Autodesk Fusion 360 part; units mm, degrees
(part 9 of 11)
  spline S8 degree 5 poles (-23.7664, -79.2655) (-23.7765, -79.2987) (-23.7959, -79.3651) (-23.8224, -79.4654) (-23.8532, -79.6002) (-23.8854, -79.7703) (-23.913, -79.9414) (-23.9379, -80.1132) (-23.9612, -80.2854) (-23.9836, -80.4578) (-24.0048, -80.6305) (-24.0246, -80.8034) (-24.0425, -80.9767) (-24.0582, -81.1505) (-24.0717, -81.3247) (-24.0832, -81.4994) (-24.0929, -81.6743) (-24.1011, -81.8495) (-24.1081, -82.0249) (-24.1139, -82.2005) (-24.1185, -82.3763) (-24.1218, -82.5523) (-24.1237, -82.7285) (-24.1243, -82.905) (-24.1235, -83.0816) (-24.1214, -83.2584) (-24.1181, -83.4354) (-24.1136, -83.6125) (-24.108, -83.7898) (-24.1013, -83.9672) (-24.0934, -84.1448) (-24.0845, -84.3225) (-24.0745, -84.5003) (-24.0634, -84.6782) (-24.0512, -84.8563) (-24.0379, -85.0344) (-24.0236, -85.2127) (-24.0082, -85.391) (-23.9919, -85.5695) (-23.9746, -85.748) (-23.9562, -85.9266) (-23.9369, -86.1053) (-23.9167, -86.2841) (-23.8955, -86.4629) (-23.8733, -86.6418) (-23.8502, -86.8207) (-23.8261, -86.9998) (-23.8011, -87.1788) (-23.7753, -87.3579) (-23.7485, -87.5371) (-23.7208, -87.7163) (-23.6922, -87.8956) (-23.6628, -88.0748) (-23.6324, -88.2541) (-23.6012, -88.4335) (-23.5692, -88.6129) (-23.5362, -88.7922) (-23.5025, -88.9717) (-23.4679, -89.1511) (-23.4324, -89.3305) (-23.3961, -89.51) (-23.359, -89.6894) (-23.3211, -89.8689) (-23.2823, -90.0484) (-23.2428, -90.2278) (-23.2024, -90.4073) (-23.1613, -90.5868) (-23.1193, -90.7662) (-23.0766, -90.9456) (-23.033, -91.1251) (-22.9887, -91.3045) (-22.9527, -91.448) (-22.9253, -91.5556) (-22.9068, -91.6274) (-22.8976, -91.6633) knots 0 0 0 0 0 0 0.01428571 0.02857143 0.04285714 0.05714286 0.07142857 0.08571429 0.1 0.11428571 0.12857143 0.14285714 0.15714286 0.17142857 0.18571429 0.2 0.21428571 0.22857143 0.24285714 0.25714286 0.27142857 0.28571429 0.3 0.31428571 0.32857143 0.34285714 0.35714286 0.37142857 0.38571429 0.4 0.41428571 0.42857143 0.44285714 0.45714286 0.47142857 0.48571429 0.5 0.51428571 0.52857143 0.54285714 0.55714286 0.57142857 0.58571429 0.6 0.61428571 0.62857143 0.64285714 0.65714286 0.67142857 0.68571429 0.7 0.71428571 0.72857143 0.74285714 0.75714286 0.77142857 0.78571429 0.8 0.81428571 0.82857143 0.84285714 0.85714286 0.87142857 0.88571429 0.9 0.91428571 0.92857143 0.94285714 0.95714286 0.97142857 0.98571429 1 1 1 1 1 1
  arc A22 (-22.8976, -91.6633) -> (-18.3724, -92.6961) centre (0.5538, 0.6546) ccw
  spline S9 degree 5 poles (-12.2104, -81.9031) (-12.2157, -81.9373) (-12.2271, -82.0056) (-12.2467, -82.1075) (-12.2774, -82.2423) (-12.3222, -82.4095) (-12.3716, -82.5757) (-12.4237, -82.7413) (-12.4774, -82.9065) (-12.5321, -83.0716) (-12.5879, -83.2363) (-12.645, -83.4007) (-12.7041, -83.5647) (-12.7654, -83.728) (-12.8288, -83.8909) (-12.8942, -84.0532) (-12.9614, -84.215) (-13.03, -84.3764) (-13.0998, -84.5375) (-13.1708, -84.6982) (-13.243, -84.8586) (-13.3164, -85.0186) (-13.3911, -85.1782) (-13.4671, -85.3374) (-13.5444, -85.4962) (-13.623, -85.6546) (-13.7028, -85.8126) (-13.7837, -85.9703) (-13.8657, -86.1276) (-13.9487, -86.2845) (-14.0328, -86.4411) (-14.118, -86.5973) (-14.2041, -86.7531) (-14.2914, -86.9086) (-14.3796, -87.0637) (-14.4689, -87.2185) (-14.5591, -87.3729) (-14.6503, -87.5269) (-14.7425, -87.6806) (-14.8355, -87.8339) (-14.9295, -87.9869) (-15.0244, -88.1395) (-15.1203, -88.2918) (-15.217, -88.4437) (-15.3146, -88.5953) (-15.4131, -88.7465) (-15.5124, -88.8973) (-15.6126, -89.0478) (-15.7136, -89.198) (-15.8155, -89.3478) (-15.9182, -89.4972) (-16.0217, -89.6463) (-16.126, -89.795) (-16.2312, -89.9434) (-16.3371, -90.0915) (-16.4438, -90.2392) (-16.5513, -90.3865) (-16.6596, -90.5335) (-16.7686, -90.6801) (-16.8784, -90.8264) (-16.9889, -90.9724) (-17.1002, -91.118) (-17.2123, -91.2632) (-17.3251, -91.4081) (-17.4386, -91.5526) (-17.5528, -91.6968) (-17.6677, -91.8406) (-17.7834, -91.9841) (-17.8998, -92.1272) (-18.0168, -92.27) (-18.1346, -92.4124) (-18.2294, -92.5261) (-18.3008, -92.6111) (-18.3485, -92.6678) (-18.3724, -92.6961) knots 0 0 0 0 0 0 0.01428571 0.02857143 0.04285714 0.05714286 0.07142857 0.08571429 0.1 0.11428571 0.12857143 0.14285714 0.15714286 0.17142857 0.18571429 0.2 0.21428571 0.22857143 0.24285714 0.25714286 0.27142857 0.28571429 0.3 0.31428571 0.32857143 0.34285714 0.35714286 0.37142857 0.38571429 0.4 0.41428571 0.42857143 0.44285714 0.45714286 0.47142857 0.48571429 0.5 0.51428571 0.52857143 0.54285714 0.55714286 0.57142857 0.58571429 0.6 0.61428571 0.62857143 0.64285714 0.65714286 0.67142857 0.68571429 0.7 0.71428571 0.72857143 0.74285714 0.75714286 0.77142857 0.78571429 0.8 0.81428571 0.82857143 0.84285714 0.85714286 0.87142857 0.88571429 0.9 0.91428571 0.92857143 0.94285714 0.95714286 0.97142857 0.98571429 1 1 1 1 1 1
  line L9 (-12.2104, -81.9031) -> (-11.9819, -80.4264)
  arc A23 (-11.0838, -79.7623) -> (-11.9819, -80.4264) centre (-11.1974, -80.5478) ccw
  arc A24 (-11.0838, -79.7623) -> (-5.9948, -80.3356) centre (0.5538, 0.6546) ccw
  arc A25 (-5.267, -81.183) -> (-5.9948, -80.3356) centre (-6.0588, -81.1268) ccw
  line L10 (-5.267, -81.183) -> (-5.3728, -82.6735)
  spline S10 degree 5 poles (-5.3728, -82.6735) (-5.3752, -82.7081) (-5.3793, -82.7772) (-5.3829, -82.8808) (-5.3829, -83.0191) (-5.3764, -83.1921) (-5.3653, -83.3651) (-5.3513, -83.5381) (-5.3357, -83.7112) (-5.3191, -83.8843) (-5.3014, -84.0573) (-5.2823, -84.2303) (-5.2612, -84.4033) (-5.2378, -84.5762) (-5.2122, -84.749) (-5.1845, -84.9218) (-5.155, -85.0946) (-5.1241, -85.2672) (-5.0918, -85.4398) (-5.0584, -85.6123) (-5.0237, -85.7847) (-4.9878, -85.957) (-4.9505, -86.1292) (-4.9118, -86.3013) (-4.8717, -86.4734) (-4.8304, -86.6453) (-4.7877, -86.8171) (-4.7439, -86.9888) (-4.699, -87.1604) (-4.653, -87.3319) (-4.6058, -87.5032) (-4.5576, -87.6745) (-4.5082, -87.8456) (-4.4578, -88.0166) (-4.4063, -88.1874) (-4.3537, -88.3582) (-4.3001, -88.5288) (-4.2454, -88.6993) (-4.1898, -88.8696) (-4.1332, -89.0398) (-4.0756, -89.2098) (-4.017, -89.3798) (-3.9575, -89.5495) (-3.897, -89.7191) (-3.8356, -89.8886) (-3.7732, -90.058) (-3.7099, -90.2271) (-3.6457, -90.3962) (-3.5806, -90.565) (-3.5147, -90.7337) (-3.4478, -90.9023) (-3.3801, -91.0707) (-3.3114, -91.2389) (-3.242, -91.407) (-3.1716, -91.5749) (-3.1005, -91.7426) (-3.0285, -91.9102) (-2.9556, -92.0776) (-2.8819, -92.2448) (-2.8074, -92.4119) (-2.7321, -92.5787) (-2.656, -92.7454) (-2.5791, -92.912) (-2.5014, -93.0783) (-2.4229, -93.2445) (-2.3436, -93.4105) (-2.2636, -93.5763) (-2.1827, -93.7419) (-2.1011, -93.9073) (-2.0188, -94.0725) (-1.9356, -94.2376) (-1.8685, -94.3695) (-1.8179, -94.4683) (-1.7839, -94.5342) (-1.7669, -94.5671) knots 0 0 0 0 0 0 0.01428571 0.02857143 0.04285714 0.05714286 0.07142857 0.08571429 0.1 0.11428571 0.12857143 0.14285714 0.15714286 0.17142857 0.18571429 0.2 0.21428571 0.22857143 0.24285714 0.25714286 0.27142857 0.28571429 0.3 0.31428571 0.32857143 0.34285714 0.35714286 0.37142857 0.38571429 0.4 0.41428571 0.42857143 0.44285714 0.45714286 0.47142857 0.48571429 0.5 0.51428571 0.52857143 0.54285714 0.55714286 0.57142857 0.58571429 0.6 0.61428571 0.62857143 0.64285714 0.65714286 0.67142857 0.68571429 0.7 0.71428571 0.72857143 0.74285714 0.75714286 0.77142857 0.78571429 0.8 0.81428571 0.82857143 0.84285714 0.85714286 0.87142857 0.88571429 0.9 0.91428571 0.92857143 0.94285714 0.95714286 0.97142857 0.98571429 1 1 1 1 1 1
  arc A26 (-1.7669, -94.5671) -> (2.8746, -94.5671) centre (0.5538, 0.6546) ccw
  spline S11 degree 5 poles (6.4805, -82.6735) (6.4829, -82.7081) (6.487, -82.7772) (6.4906, -82.8808) (6.4906, -83.0191) (6.4841, -83.1921) (6.473, -83.3651) (6.459, -83.5381) (6.4434, -83.7112) (6.4268, -83.8843) (6.4091, -84.0573) (6.39, -84.2303) (6.3689, -84.4033) (6.3455, -84.5762) (6.3199, -84.749) (6.2922, -84.9218) (6.2627, -85.0946) (6.2318, -85.2672) (6.1995, -85.4398) (6.1661, -85.6123) (6.1314, -85.7847) (6.0955, -85.957) (6.0582, -86.1292) (6.0195, -86.3013) (5.9794, -86.4734) (5.9381, -86.6453) (5.8954, -86.8171) (5.8516, -86.9888) (5.8067, -87.1604) (5.7607, -87.3319) (5.7135, -87.5032) (5.6653, -87.6745) (5.6159, -87.8456) (5.5655, -88.0166) (5.514, -88.1874) (5.4614, -88.3582) (5.4078, -88.5288) (5.3531, -88.6993) (5.2975, -88.8696) (5.2409, -89.0398) (5.1833, -89.2098) (5.1247, -89.3798) (5.0652, -89.5495) (5.0047, -89.7191) (4.9432, -89.8886) (4.8809, -90.058) (4.8176, -90.2271) (4.7534, -90.3962) (4.6883, -90.565) (4.6223, -90.7337) (4.5555, -90.9023) (4.4877, -91.0707) (4.4191, -91.2389) (4.3497, -91.407) (4.2793, -91.5749) (4.2082, -91.7426) (4.1361, -91.9102) (4.0633, -92.0776) (3.9896, -92.2448) (3.9151, -92.4119) (3.8398, -92.5787) (3.7637, -92.7454) (3.6868, -92.912) (3.6091, -93.0783) (3.5306, -93.2445) (3.4513, -93.4105) (3.3712, -93.5763) (3.2904, -93.7419) (3.2088, -93.9073) (3.1264, -94.0725) (3.0433, -94.2376) (2.9762, -94.3695) (2.9255, -94.4683) (2.8916, -94.5342) (2.8746, -94.5671) knots 0 0 0 0 0 0 0.01428571 0.02857143 0.04285714 0.05714286 0.07142857 0.08571429 0.1 0.11428571 0.12857143 0.14285714 0.15714286 0.17142857 0.18571429 0.2 0.21428571 0.22857143 0.24285714 0.25714286 0.27142857 0.28571429 0.3 0.31428571 0.32857143 0.34285714 0.35714286 0.37142857 0.38571429 0.4 0.41428571 0.42857143 0.44285714 0.45714286 0.47142857 0.48571429 0.5 0.51428571 0.52857143 0.54285714 0.55714286 0.57142857 0.58571429 0.6 0.61428571 0.62857143 0.64285714 0.65714286 0.67142857 0.68571429 0.7 0.71428571 0.72857143 0.74285714 0.75714286 0.77142857 0.78571429 0.8 0.81428571 0.82857143 0.84285714 0.85714286 0.87142857 0.88571429 0.9 0.91428571 0.92857143 0.94285714 0.95714286 0.97142857 0.98571429 1 1 1 1 1 1
  line L11 (6.4805, -82.6735) -> (6.3747, -81.183)
  arc A27 (7.1025, -80.3356) -> (6.3747, -81.183) centre (7.1664, -81.1268) ccw
  arc A28 (7.1025, -80.3356) -> (12.1914, -79.7623) centre (0.5538, 0.6546) ccw
  arc A29 (13.0895, -80.4264) -> (12.1914, -79.7623) centre (12.3051, -80.5478) ccw
  line L12 (13.0895, -80.4264) -> (13.3181, -81.9031)
  spline S12 degree 5 poles (13.3181, -81.9031) (13.3234, -81.9373) (13.3348, -82.0056) (13.3544, -82.1075) (13.3851, -82.2423) (13.4299, -82.4095) (13.4793, -82.5757) (13.5314, -82.7413) (13.5851, -82.9065) (13.6398, -83.0716) (13.6955, -83.2363) (13.7527, -83.4007) (13.8118, -83.5647) (13.873, -83.728) (13.9365, -83.8909) (14.0019, -84.0532) (14.0691, -84.215) (14.1377, -84.3764) (14.2075, -84.5375) (14.2785, -84.6982) (14.3507, -84.8586) (14.424, -85.0186) (14.4987, -85.1782) (14.5748, -85.3374) (14.6521, -85.4962) (14.7307, -85.6546) (14.8105, -85.8126) (14.8914, -85.9703) (14.9734, -86.1276) (15.0564, -86.2845) (15.1405, -86.4411) (15.2256, -86.5973) (15.3118, -86.7531) (15.399, -86.9086) (15.4873, -87.0637) (15.5766, -87.2185) (15.6668, -87.3729) (15.758, -87.5269) (15.8501, -87.6806) (15.9432, -87.8339) (16.0372, -87.9869) (16.1321, -88.1395) (16.2279, -88.2918) (16.3247, -88.4437) (16.4223, -88.5953) (16.5207, -88.7465) (16.6201, -88.8973) (16.7203, -89.0478) (16.8213, -89.198) (16.9232, -89.3478) (17.0259, -89.4972) (17.1294, -89.6463) (17.2337, -89.795) (17.3388, -89.9434) (17.4448, -90.0915) (17.5515, -90.2392) (17.659, -90.3865) (17.7672, -90.5335) (17.8763, -90.6801) (17.9861, -90.8264) (18.0966, -90.9724) (18.2079, -91.118) (18.32, -91.2632) (18.4327, -91.4081) (18.5462, -91.5526) (18.6605, -91.6968) (18.7754, -91.8406) (18.8911, -91.9841) (19.0075, -92.1272) (19.1245, -92.27) (19.2423, -92.4124) (19.3371, -92.5261) (19.4084, -92.6111) (19.4562, -92.6678) (19.4801, -92.6961) knots 0 0 0 0 0 0 0.01428571 0.02857143 0.04285714 0.05714286 0.07142857 0.08571429 0.1 0.11428571 0.12857143 0.14285714 0.15714286 0.17142857 0.18571429 0.2 0.21428571 0.22857143 0.24285714 0.25714286 0.27142857 0.28571429 0.3 0.31428571 0.32857143 0.34285714 0.35714286 0.37142857 0.38571429 0.4 0.41428571 0.42857143 0.44285714 0.45714286 0.47142857 0.48571429 0.5 0.51428571 0.52857143 0.54285714 0.55714286 0.57142857 0.58571429 0.6 0.61428571 0.62857143 0.64285714 0.65714286 0.67142857 0.68571429 0.7 0.71428571 0.72857143 0.74285714 0.75714286 0.77142857 0.78571429 0.8 0.81428571 0.82857143 0.84285714 0.85714286 0.87142857 0.88571429 0.9 0.91428571 0.92857143 0.94285714 0.95714286 0.97142857 0.98571429 1 1 1 1 1 1
  arc A30 (19.4801, -92.6961) -> (24.0053, -91.6633) centre (0.5538, 0.6546) ccw
  spline S13 degree 5 poles (24.8741, -79.2655) (24.8842, -79.2987) (24.9035, -79.3651) (24.9301, -79.4654) (24.9609, -79.6002) (24.9931, -79.7703) (25.0207, -79.9414) (25.0456, -80.1132) (25.0689, -80.2854) (25.0912, -80.4578) (25.1125, -80.6305) (25.1323, -80.8034) (25.1502, -80.9767) (25.1659, -81.1505) (25.1794, -81.3247) (25.1909, -81.4994) (25.2006, -81.6743) (25.2088, -81.8495) (25.2158, -82.0249) (25.2216, -82.2005) (25.2261, -82.3763) (25.2294, -82.5523) (25.2314, -82.7285) (25.232, -82.905) (25.2312, -83.0816) (25.2291, -83.2584) (25.2258, -83.4354) (25.2213, -83.6125) (25.2157, -83.7898) (25.209, -83.9672) (25.2011, -84.1448) (25.1922, -84.3225) (25.1822, -84.5003) (25.171, -84.6782) (25.1588, -84.8563) (25.1456, -85.0344) (25.1312, -85.2127) (25.1159, -85.391) (25.0996, -85.5695) (25.0822, -85.748) (25.0639, -85.9266) (25.0446, -86.1053) (25.0244, -86.2841) (25.0031, -86.4629) (24.981, -86.6418) (24.9578, -86.8207) (24.9338, -86.9998) (24.9088, -87.1788) (24.8829, -87.3579) (24.8562, -87.5371) (24.8285, -87.7163) (24.7999, -87.8956) (24.7705, -88.0748) (24.7401, -88.2541) (24.7089, -88.4335) (24.6769, -88.6129) (24.6439, -88.7922) (24.6102, -88.9717) (24.5755, -89.1511) (24.5401, -89.3305) (24.5038, -89.51) (24.4667, -89.6894) (24.4288, -89.8689) (24.39, -90.0484) (24.3505, -90.2278) (24.3101, -90.4073) (24.2689, -90.5868) (24.227, -90.7662) (24.1843, -90.9456) (24.1407, -91.1251) (24.0964, -91.3045) (24.0603, -91.448) (24.0329, -91.5556) (24.0145, -91.6274) (24.0053, -91.6633) knots 0 0 0 0 0 0 0.01428571 0.02857143 0.04285714 0.05714286 0.07142857 0.08571429 0.1 0.11428571 0.12857143 0.14285714 0.15714286 0.17142857 0.18571429 0.2 0.21428571 0.22857143 0.24285714 0.25714286 0.27142857 0.28571429 0.3 0.31428571 0.32857143 0.34285714 0.35714286 0.37142857 0.38571429 0.4 0.41428571 0.42857143 0.44285714 0.45714286 0.47142857 0.48571429 0.5 0.51428571 0.52857143 0.54285714 0.55714286 0.57142857 0.58571429 0.6 0.61428571 0.62857143 0.64285714 0.65714286 0.67142857 0.68571429 0.7 0.71428571 0.72857143 0.74285714 0.75714286 0.77142857 0.78571429 0.8 0.81428571 0.82857143 0.84285714 0.85714286 0.87142857 0.88571429 0.9 0.91428571 0.92857143 0.94285714 0.95714286 0.97142857 0.98571429 1 1 1 1 1 1
  line L13 (24.8741, -79.2655) -> (24.4393, -77.8359)
  arc A31 (24.9603, -76.8478) -> (24.4393, -77.8359) centre (25.1987, -77.6049) ccw
  arc A32 (24.9603, -76.8478) -> (29.7941, -75.1564) centre (0.5538, 0.6546) ccw
  arc A33 (30.8175, -75.6041) -> (29.7941, -75.1564) centre (30.0797, -75.897) ccw
  line L14 (30.8175, -75.6041) -> (31.3689, -76.9929)
  spline S14 degree 5 poles (31.3689, -76.9929) (31.3817, -77.0251) (31.408, -77.0891) (31.4497, -77.1841) (31.5097, -77.3087) (31.5906, -77.4617) (31.6757, -77.6127) (31.7634, -77.7626) (31.8525, -77.9118) (31.9425, -78.0605) (32.0336, -78.2087) (32.1259, -78.3563) (32.2199, -78.5029) (32.316, -78.6486) (32.4141, -78.7932) (32.514, -78.9369) (32.6155, -79.0797) (32.7183, -79.2218) (32.8222, -79.3633) (32.9272, -79.5042) (33.0332, -79.6445) (33.1404, -79.7842) (33.2487, -79.9232) (33.3583, -80.0615) (33.469, -80.1991) (33.5809, -80.336) (33.6938, -80.4723) (33.8078, -80.608) (33.9227, -80.7431) (34.0386, -80.8776) (34.1554, -81.0116) (34.2732, -81.1449) (34.3919, -81.2777) (34.5115, -81.4098) (34.6321, -81.5414) (34.7535, -81.6724) (34.8758, -81.8029) (34.999, -81.9328) (35.1231, -82.0621) (35.2479, -82.1909) (35.3736, -82.3191) (35.5001, -82.4468) (35.6274, -82.5739) (35.7555, -82.7005) (35.8844, -82.8265) (36.014, -82.952) (36.1444, -83.077) (36.2756, -83.2014) (36.4075, -83.3253) (36.5402, -83.4487) (36.6735, -83.5715) (36.8076, -83.6939) (36.9425, -83.8157) (37.078, -83.9369) (37.2142, -84.0577) (37.3511, -84.178) (37.4887, -84.2977) (37.6269, -84.4169) (37.7659, -84.5356) (37.9055, -84.6538) (38.0457, -84.7715) (38.1866, -84.8886) (38.3282, -85.0053) (38.4704, -85.1214) (38.6132, -85.2371) (38.7566, -85.3522) (38.9007, -85.4669) (39.0454, -85.581) (39.1907, -85.6947) (39.3366, -85.8078) (39.4831, -85.9205) (39.6008, -86.0102) (39.6893, -86.0772) (39.7485, -86.1218) (39.7781, -86.1441) knots 0 0 0 0 0 0 0.01428571 0.02857143 0.04285714 0.05714286 0.07142857 0.08571429 0.1 0.11428571 0.12857143 0.14285714 0.15714286 0.17142857 0.18571429 0.2 0.21428571 0.22857143 0.24285714 0.25714286 0.27142857 0.28571429 0.3 0.31428571 0.32857143 0.34285714 0.35714286 0.37142857 0.38571429 0.4 0.41428571 0.42857143 0.44285714 0.45714286 0.47142857 0.48571429 0.5 0.51428571 0.52857143 0.54285714 0.55714286 0.57142857 0.58571429 0.6 0.61428571 0.62857143 0.64285714 0.65714286 0.67142857 0.68571429 0.7 0.71428571 0.72857143 0.74285714 0.75714286 0.77142857 0.78571429 0.8 0.81428571 0.82857143 0.84285714 0.85714286 0.87142857 0.88571429 0.9 0.91428571 0.92857143 0.94285714 0.95714286 0.97142857 0.98571429 1 1 1 1 1 1
  arc A34 (39.7781, -86.1441) -> (43.9599, -84.1302) centre (0.5538, 0.6546) ccw
  spline S15 degree 5 poles (42.0483, -71.85) (42.0655, -71.88) (42.0991, -71.9405) (42.1473, -72.0324) (42.2074, -72.157) (42.2766, -72.3156) (42.3416, -72.4763) (42.4041, -72.6383) (42.4651, -72.801) (42.5253, -72.9641) (42.5844, -73.1277) (42.6422, -73.2919) (42.6982, -73.4569) (42.7522, -73.6228) (42.8041, -73.7896) (42.8542, -73.9573) (42.9025, -74.1257) (42.9496, -74.2947) (42.9954, -74.4642) (43.0401, -74.6341) (43.0837, -74.8045) (43.1261, -74.9753) (43.1672, -75.1467) (43.207, -75.3185) (43.2456, -75.4909) (43.2829, -75.6638) (43.319, -75.8371) (43.354, -76.0108) (43.388, -76.1848) (43.4209, -76.3593) (43.4528, -76.5342) (43.4836, -76.7094) (43.5134, -76.885) (43.5422, -77.0609) (43.5699, -77.2372) (43.5966, -77.4138) (43.6223, -77.5908) (43.6471, -77.7681) (43.6708, -77.9457) (43.6937, -78.1236) (43.7155, -78.3018) (43.7365, -78.4803) (43.7565, -78.6591) (43.7756, -78.8382) (43.7938, -79.0175) (43.8111, -79.1971) (43.8275, -79.377) (43.843, -79.5572) (43.8576, -79.7375) (43.8714, -79.9182) (43.8842, -80.0991) (43.8963, -80.2802) (43.9075, -80.4615) (43.9178, -80.6431) (43.9273, -80.8249) (43.9359, -81.0069) (43.9437, -81.1891) (43.9507, -81.3715) (43.9569, -81.5541) (43.9623, -81.737) (43.9669, -81.92) (43.9706, -82.1032) (43.9736, -82.2866) (43.9757, -82.4702) (43.9771, -82.654) (43.9777, -82.8379) (43.9775, -83.022) (43.9765, -83.2063) (43.9748, -83.3908) (43.9723, -83.5754) (43.969, -83.7602) (43.9657, -83.9081) (43.963, -84.0191) (43.961, -84.0932) (43.9599, -84.1302) knots 0 0 0 0 0 0 0.01428571 0.02857143 0.04285714 0.05714286 0.07142857 0.08571429 0.1 0.11428571 0.12857143 0.14285714 0.15714286 0.17142857 0.18571429 0.2 0.21428571 0.22857143 0.24285714 0.25714286 0.27142857 0.28571429 0.3 0.31428571 0.32857143 0.34285714 0.35714286 0.37142857 0.38571429 0.4 0.41428571 0.42857143 0.44285714 0.45714286 0.47142857 0.48571429 0.5 0.51428571 0.52857143 0.54285714 0.55714286 0.57142857 0.58571429 0.6 0.61428571 0.62857143 0.64285714 0.65714286 0.67142857 0.68571429 0.7 0.71428571 0.72857143 0.74285714 0.75714286 0.77142857 0.78571429 0.8 0.81428571 0.82857143 0.84285714 0.85714286 0.87142857 0.88571429 0.9 0.91428571 0.92857143 0.94285714 0.95714286 0.97142857 0.98571429 1 1 1 1 1 1
  line L15 (42.0483, -71.85) -> (41.3063, -70.553)
  arc A35 (41.5943, -69.4737) -> (41.3063, -70.553) centre (41.9952, -70.1588) ccw
  arc A36 (41.5943, -69.4737) -> (45.9305, -66.7491) centre (0.5538, 0.6546) ccw
  arc A37 (47.0279, -66.9578) -> (45.9305, -66.7491) centre (46.3738, -67.4076) ccw
  line L16 (47.0279, -66.9578) -> (47.8745, -68.1891)
  spline S16 degree 5 poles (47.8745, -68.1891) (47.8941, -68.2177) (47.934, -68.2742) (47.9958, -68.3575) (48.082, -68.4657) (48.1949, -68.5968) (48.3115, -68.7252) (48.4304, -68.8517) (48.5504, -68.9773) (48.6713, -69.1023) (48.793, -69.2265) (48.9159, -69.3498) (49.0402, -69.4719) (49.1663, -69.5925) (49.2941, -69.7117) (49.4235, -69.8295) (49.5542, -69.9462) (49.6861, -70.0619) (49.8189, -70.1767) (49.9526, -70.2907) (50.0871, -70.4039) (50.2227, -70.5162) (50.3592, -70.6276) (50.4968, -70.7381) (50.6354, -70.8476) (50.7749, -70.9562) (50.9154, -71.0639) (51.0567, -71.1709) (51.1988, -71.277) (51.3417, -71.3824) (51.4854, -71.487) (51.6299, -71.5908) (51.7751, -71.6938) (51.9212, -71.796) (52.068, -71.8975) (52.2156, -71.9982) (52.3638, -72.0981) (52.5129, -72.1974) (52.6626, -72.2958) (52.8129, -72.3936) (52.964, -72.4906) (53.1157, -72.587) (53.2681, -72.6826) (53.4212, -72.7775) (53.5749, -72.8717) (53.7292, -72.9652) (53.8842, -73.058) (54.0397, -73.1501) (54.1959, -73.2416) (54.3527, -73.3323) (54.51, -73.4224) (54.668, -73.5118) (54.8265, -73.6006) (54.9856, -73.6887) (55.1453, -73.7761) (55.3055, -73.8629) (55.4663, -73.949) (55.6276, -74.0344) (55.7895, -74.1192) (55.9519, -74.2034) (56.1148, -74.2869) (56.2783, -74.3698) (56.4422, -74.452) (56.6067, -74.5336) (56.7717, -74.6146) (56.9371, -74.695) (57.1031, -74.7747) (57.2696, -74.8537) (57.4365, -74.9322) (57.6039, -75.01) (57.7718, -75.0873) (57.9065, -75.1485) (58.0078, -75.1942) (58.0753, -75.2245) (58.1092, -75.2397) knots 0 0 0 0 0 0 0.01428571 0.02857143 0.04285714 0.05714286 0.07142857 0.08571429 0.1 0.11428571 0.12857143 0.14285714 0.15714286 0.17142857 0.18571429 0.2 0.21428571 0.22857143 0.24285714 0.25714286 0.27142857 0.28571429 0.3 0.31428571 0.32857143 0.34285714 0.35714286 0.37142857 0.38571429 0.4 0.41428571 0.42857143 0.44285714 0.45714286 0.47142857 0.48571429 0.5 0.51428571 0.52857143 0.54285714 0.55714286 0.57142857 0.58571429 0.6 0.61428571 0.62857143 0.64285714 0.65714286 0.67142857 0.68571429 0.7 0.71428571 0.72857143 0.74285714 0.75714286 0.77142857 0.78571429 0.8 0.81428571 0.82857143 0.84285714 0.85714286 0.87142857 0.88571429 0.9 0.91428571 0.92857143 0.94285714 0.95714286 0.97142857 0.98571429 1 1 1 1 1 1
  arc A38 (58.1092, -75.2397) -> (61.7381, -72.3457) centre (0.5538, 0.6546) ccw
  spline S17 degree 5 poles (57.1417, -60.7988) (57.1652, -60.8242) (57.2114, -60.8757) (57.2789, -60.9545) (57.3651, -61.0626) (57.4679, -61.2019) (57.5671, -61.3441) (57.664, -61.4881) (57.7597, -61.6331) (57.8547, -61.7788) (57.9487, -61.9251) (58.0416, -62.0723) (58.1329, -62.2207) (58.2225, -62.3705) (58.3102, -62.5216) (58.3963, -62.6739) (58.481, -62.8274) (58.5644, -62.9817) (58.6468, -63.1367) (58.7282, -63.2924) (58.8086, -63.4488) (58.8879, -63.6059) (58.9662, -63.7638) (59.0432, -63.9225) (59.1192, -64.082) (59.194, -64.2422) (59.2678, -64.4031) (59.3406, -64.5647) (59.4125, -64.7268) (59.4834, -64.8896) (59.5534, -65.053) (59.6224, -65.2169) (59.6905, -65.3815) (59.7577, -65.5466) (59.824, -65.7123) (59.8893, -65.8786) (59.9537, -66.0454) (60.0173, -66.2127) (60.08, -66.3806) (60.1419, -66.549) (60.2029, -66.7178) (60.263, -66.8872) (60.3223, -67.0571) (60.3808, -67.2274) (60.4384, -67.3982) (60.4952, -67.5695) (60.5512, -67.7412) (60.6064, -67.9133) (60.6608, -68.086) (60.7144, -68.259) (60.7673, -68.4325) (60.8193, -68.6064) (60.8705, -68.7807) (60.921, -68.9554) (60.9707, -69.1305) (61.0196, -69.306) (61.0678, -69.4819) (61.1152, -69.6582) (61.1619, -69.8349) (61.2078, -70.0119) (61.253, -70.1894) (61.2974, -70.3672) (61.3411, -70.5453) (61.3841, -70.7238) (61.4263, -70.9027) (61.4678, -71.0819) (61.5086, -71.2614) (61.5486, -71.4413) (61.588, -71.6215) (61.6266, -71.8021) (61.6645, -71.9829) (61.6943, -72.1279) (61.7163, -72.2367) (61.7308, -72.3094) (61.7381, -72.3457) knots 0 0 0 0 0 0 0.01428571 0.02857143 0.04285714 0.05714286 0.07142857 0.08571429 0.1 0.11428571 0.12857143 0.14285714 0.15714286 0.17142857 0.18571429 0.2 0.21428571 0.22857143 0.24285714 0.25714286 0.27142857 0.28571429 0.3 0.31428571 0.32857143 0.34285714 0.35714286 0.37142857 0.38571429 0.4 0.41428571 0.42857143 0.44285714 0.45714286 0.47142857 0.48571429 0.5 0.51428571 0.52857143 0.54285714 0.55714286 0.57142857 0.58571429 0.6 0.61428571 0.62857143 0.64285714 0.65714286 0.67142857 0.68571429 0.7 0.71428571 0.72857143 0.74285714 0.75714286 0.77142857 0.78571429 0.8 0.81428571 0.82857143 0.84285714 0.85714286 0.87142857 0.88571429 0.9 0.91428571 0.92857143 0.94285714 0.95714286 0.97142857 0.98571429 1 1 1 1 1 1
  line L17 (57.1417, -60.7988) -> (56.1297, -59.6994)
  arc A39 (56.1704, -58.5831) -> (56.1297, -59.6994) centre (56.7137, -59.1618) ccw
  arc A40 (56.1704, -58.5831) -> (59.7916, -54.9619) centre (0.5538, 0.6546) ccw
  arc A41 (60.9079, -54.9212) -> (59.7916, -54.9619) centre (60.3703, -55.5052) ccw
  line L18 (60.9079, -54.9212) -> (62.0072, -55.9332)
  spline S18 degree 5 poles (62.0072, -55.9332) (62.0327, -55.9567) (62.0842, -56.003) (62.163, -56.0704) (62.2711, -56.1566) (62.4104, -56.2594) (62.5526, -56.3586) (62.6966, -56.4555) (62.8416, -56.5513) (62.9873, -56.6462) (63.1336, -56.7402) (63.2808, -56.8331) (63.4292, -56.9245) (63.579, -57.014) (63.7301, -57.1018) (63.8824, -57.1878) (64.0358, -57.2725) (64.1901, -57.3559) (64.3452, -57.4383) (64.5009, -57.5197) (64.6573, -57.6001) (64.8144, -57.6795) (64.9723, -57.7577) (65.131, -57.8347) (65.2905, -57.9107) (65.4507, -57.9855) (65.6116, -58.0593) (65.7731, -58.1321) (65.9353, -58.204) (66.0981, -58.2749) (66.2614, -58.3449) (66.4254, -58.4139) (66.5899, -58.4821) (66.7551, -58.5492) (66.9208, -58.6155) (67.0871, -58.6808) (67.2539, -58.7453) (67.4212, -58.8088) (67.5891, -58.8715) (67.7575, -58.9334) (67.9263, -58.9944) (68.0957, -59.0545) (68.2655, -59.1138) (68.4359, -59.1723) (68.6067, -59.2299) (68.7779, -59.2868) (68.9497, -59.3428) (69.1218, -59.398) (69.2944, -59.4524) (69.4675, -59.506) (69.6409, -59.5588) (69.8148, -59.6108) (69.9891, -59.662) (70.1639, -59.7125) (70.339, -59.7622) (70.5145, -59.8112) (70.6904, -59.8593) (70.8667, -59.9067) (71.0434, -59.9534) (71.2204, -59.9993) (71.3978, -60.0445) (71.5756, -60.0889) (71.7538, -60.1326) (71.9323, -60.1756) (72.1112, -60.2178) (72.2904, -60.2593) (72.4699, -60.3001) (72.6498, -60.3402) (72.83, -60.3795) (73.0105, -60.4181) (73.1914, -60.4561) (73.3364, -60.4858) (73.4452, -60.5078) (73.5179, -60.5224) (73.5542, -60.5296) knots 0 0 0 0 0 0 0.01428571 0.02857143 0.04285714 0.05714286 0.07142857 0.08571429 0.1 0.11428571 0.12857143 0.14285714 0.15714286 0.17142857 0.18571429 0.2 0.21428571 0.22857143 0.24285714 0.25714286 0.27142857 0.28571429 0.3 0.31428571 0.32857143 0.34285714 0.35714286 0.37142857 0.38571429 0.4 0.41428571 0.42857143 0.44285714 0.45714286 0.47142857 0.48571429 0.5 0.51428571 0.52857143 0.54285714 0.55714286 0.57142857 0.58571429 0.6 0.61428571 0.62857143 0.64285714 0.65714286 0.67142857 0.68571429 0.7 0.71428571 0.72857143 0.74285714 0.75714286 0.77142857 0.78571429 0.8 0.81428571 0.82857143 0.84285714 0.85714286 0.87142857 0.88571429 0.9 0.91428571 0.92857143 0.94285714 0.95714286 0.97142857 0.98571429 1 1 1 1 1 1
  arc A42 (73.5542, -60.5296) -> (76.4482, -56.9007) centre (0.5538, 0.6546) ccw
  spline S19 degree 5 poles (69.3976, -46.666) (69.4262, -46.6856) (69.4827, -46.7255) (69.566, -46.7874) (69.6741, -46.8736) (69.8053, -46.9865) (69.9336, -47.103) (70.0602, -47.2219) (70.1858, -47.342) (70.3108, -47.4628) (70.435, -47.5846) (70.5583, -47.7074) (70.6804, -47.8317) (70.801, -47.9578) (70.9202, -48.0856) (71.038, -48.215) (71.1547, -48.3457) (71.2704, -48.4776) (71.3852, -48.6104) (71.4992, -48.7441) (71.6124, -48.8787) (71.7247, -49.0142) (71.8361, -49.1508) (71.9465, -49.2883) (72.0561, -49.4269) (72.1647, -49.5664) (72.2724, -49.7069) (72.3794, -49.8482) (72.4855, -49.9903) (72.5909, -50.1332) (72.6954, -50.2769) (72.7992, -50.4214) (72.9023, -50.5667) (73.0045, -50.7127) (73.106, -50.8595) (73.2067, -51.0071) (73.3066, -51.1554) (73.4058, -51.3044) (73.5043, -51.4541) (73.6021, -51.6045) (73.6991, -51.7555) (73.7954, -51.9073) (73.8911, -52.0596) (73.986, -52.2127) (74.0802, -52.3664) (74.1737, -52.5207) (74.2665, -52.6757) (74.3586, -52.8312) (74.45, -52.9874) (74.5408, -53.1442) (74.6309, -53.3016) (74.7203, -53.4595) (74.8091, -53.618) (74.8972, -53.7772) (74.9846, -53.9368) (75.0713, -54.097) (75.1575, -54.2578) (75.2429, -54.4191) (75.3277, -54.581) (75.4119, -54.7434) (75.4954, -54.9063) (75.5783, -55.0698) (75.6605, -55.2337) (75.7421, -55.3982) (75.8231, -55.5632) (75.9034, -55.7287) (75.9831, -55.8946) (76.0622, -56.0611) (76.1407, -56.228) (76.2185, -56.3954) (76.2957, -56.5633) (76.357, -56.698) (76.4027, -56.7993) (76.433, -56.8669) (76.4482, -56.9007) knots 0 0 0 0 0 0 0.01428571 0.02857143 0.04285714 0.05714286 0.07142857 0.08571429 0.1 0.11428571 0.12857143 0.14285714 0.15714286 0.17142857 0.18571429 0.2 0.21428571 0.22857143 0.24285714 0.25714286 0.27142857 0.28571429 0.3 0.31428571 0.32857143 0.34285714 0.35714286 0.37142857 0.38571429 0.4 0.41428571 0.42857143 0.44285714 0.45714286 0.47142857 0.48571429 0.5 0.51428571 0.52857143 0.54285714 0.55714286 0.57142857 0.58571429 0.6 0.61428571 0.62857143 0.64285714 0.65714286 0.67142857 0.68571429 0.7 0.71428571 0.72857143 0.74285714 0.75714286 0.77142857 0.78571429 0.8 0.81428571 0.82857143 0.84285714 0.85714286 0.87142857 0.88571429 0.9 0.91428571 0.92857143 0.94285714 0.95714286 0.97142857 0.98571429 1 1 1 1 1 1
  line L19 (69.3976, -46.666) -> (68.1663, -45.8194)
  arc A43 (67.9576, -44.7221) -> (68.1663, -45.8194) centre (68.616, -45.1653) ccw
  arc A44 (67.9576, -44.7221) -> (70.6822, -40.3858) centre (0.5538, 0.6546) ccw
  arc A45 (71.7614, -40.0978) -> (70.6822, -40.3858) centre (71.3673, -40.7867) ccw
  line L20 (71.7614, -40.0978) -> (73.0585, -40.8398)
  spline S20 degree 5 poles (73.0585, -40.8398) (73.0885, -40.857) (73.149, -40.8906) (73.2409, -40.9389) (73.3654, -40.9989) (73.5241, -41.0681) (73.6848, -41.1331) (73.8468, -41.1956) (74.0095, -41.2566) (74.1726, -41.3168) (74.3362, -41.3759) (74.5003, -41.4337) (74.6653, -41.4898) (74.8313, -41.5437) (74.9981, -41.5957) (75.1658, -41.6457) (75.3342, -41.6941) (75.5032, -41.7411) (75.6727, -41.7869) (75.8426, -41.8316) (76.013, -41.8752) (76.1838, -41.9176) (76.3552, -41.9587) (76.527, -41.9985) (76.6994, -42.0371) (76.8722, -42.0744) (77.0455, -42.1105) (77.2192, -42.1456) (77.3933, -42.1795) (77.5678, -42.2125) (77.7426, -42.2443) (77.9179, -42.2752) (78.0934, -42.305) (78.2694, -42.3337) (78.4457, -42.3614) (78.6223, -42.3881) (78.7993, -42.4138) (78.9766, -42.4386) (79.1542, -42.4623) (79.3321, -42.4852) (79.5103, -42.5071) (79.6888, -42.528) (79.8676, -42.548) (80.0467, -42.5671) (80.226, -42.5853) (80.4056, -42.6026) (80.5855, -42.619) (80.7656, -42.6345) (80.946, -42.6491) (81.1267, -42.6629) (81.3075, -42.6758) (81.4886, -42.6878) (81.67, -42.699) (81.8515, -42.7093) (82.0333, -42.7188) (82.2153, -42.7274) (82.3976, -42.7353) (82.58, -42.7423) (82.7626, -42.7484) (82.9454, -42.7538) (83.1285, -42.7584) (83.3117, -42.7621) (83.4951, -42.7651) (83.6787, -42.7672) (83.8625, -42.7686) (84.0464, -42.7692) (84.2305, -42.769) (84.4148, -42.768) (84.5993, -42.7663) (84.7839, -42.7638) (84.9686, -42.7605) (85.1166, -42.7573) (85.2276, -42.7545) (85.3017, -42.7525) (85.3387, -42.7515) knots 0 0 0 0 0 0 0.01428571 0.02857143 0.04285714 0.05714286 0.07142857 0.08571429 0.1 0.11428571 0.12857143 0.14285714 0.15714286 0.17142857 0.18571429 0.2 0.21428571 0.22857143 0.24285714 0.25714286 0.27142857 0.28571429 0.3 0.31428571 0.32857143 0.34285714 0.35714286 0.37142857 0.38571429 0.4 0.41428571 0.42857143 0.44285714 0.45714286 0.47142857 0.48571429 0.5 0.51428571 0.52857143 0.54285714 0.55714286 0.57142857 0.58571429 0.6 0.61428571 0.62857143 0.64285714 0.65714286 0.67142857 0.68571429 0.7 0.71428571 0.72857143 0.74285714 0.75714286 0.77142857 0.78571429 0.8 0.81428571 0.82857143 0.84285714 0.85714286 0.87142857 0.88571429 0.9 0.91428571 0.92857143 0.94285714 0.95714286 0.97142857 0.98571429 1 1 1 1 1 1
  arc A46 (85.3387, -42.7515) -> (87.3526, -38.5696) centre (0.5538, 0.6546) ccw
  spline S21 degree 5 poles (78.2014, -30.1604) (78.2336, -30.1732) (78.2976, -30.1995) (78.3926, -30.2412) (78.5172, -30.3012) (78.6702, -30.3821) (78.8212, -30.4672) (78.9711, -30.5549) (79.1202, -30.644) (79.269, -30.7341) (79.4172, -30.8251) (79.5647, -30.9174) (79.7114, -31.0115) (79.8571, -31.1075) (80.0017, -31.2056) (80.1454, -31.3055) (80.2882, -31.407) (80.4303, -31.5098) (80.5718, -31.6138) (80.7127, -31.7187) (80.853, -31.8248) (80.9927, -31.9319) (81.1316, -32.0402) (81.2699, -32.1498) (81.4075, -32.2605) (81.5445, -32.3724) (81.6808, -32.4853) (81.8165, -32.5993) (81.9516, -32.7142) (82.0861, -32.8301) (82.22, -32.9469) (82.3534, -33.0647) (82.4862, -33.1834) (82.6183, -33.303) (82.7499, -33.4236) (82.8809, -33.545) (83.0114, -33.6674) (83.1413, -33.7906) (83.2706, -33.9146) (83.3993, -34.0395) (83.5276, -34.1651) (83.6552, -34.2916) (83.7824, -34.4189) (83.909, -34.547) (84.035, -34.6759) (84.1605, -34.8055) (84.2855, -34.936) (84.4099, -35.0671) (84.5338, -35.199) (84.6572, -35.3317) (84.78, -35.4651) (84.9023, -35.5992) (85.0241, -35.734) (85.1454, -35.8695) (85.2662, -36.0057) (85.3864, -36.1426) (85.5062, -36.2802) (85.6254, -36.4185) (85.7441, -36.5574) (85.8623, -36.697) (85.9799, -36.8372) (86.0971, -36.9781) (86.2138, -37.1197) (86.3299, -37.2619) (86.4456, -37.4047) (86.5607, -37.5482) (86.6754, -37.6922) (86.7895, -37.8369) (86.9032, -37.9822) (87.0163, -38.1281) (87.1289, -38.2746) (87.2186, -38.3923) (87.2857, -38.4808) (87.3303, -38.54) (87.3526, -38.5696) knots 0 0 0 0 0 0 0.01428571 0.02857143 0.04285714 0.05714286 0.07142857 0.08571429 0.1 0.11428571 0.12857143 0.14285714 0.15714286 0.17142857 0.18571429 0.2 0.21428571 0.22857143 0.24285714 0.25714286 0.27142857 0.28571429 0.3 0.31428571 0.32857143 0.34285714 0.35714286 0.37142857 0.38571429 0.4 0.41428571 0.42857143 0.44285714 0.45714286 0.47142857 0.48571429 0.5 0.51428571 0.52857143 0.54285714 0.55714286 0.57142857 0.58571429 0.6 0.61428571 0.62857143 0.64285714 0.65714286 0.67142857 0.68571429 0.7 0.71428571 0.72857143 0.74285714 0.75714286 0.77142857 0.78571429 0.8 0.81428571 0.82857143 0.84285714 0.85714286 0.87142857 0.88571429 0.9 0.91428571 0.92857143 0.94285714 0.95714286 0.97142857 0.98571429 1 1 1 1 1 1
  line L21 (78.2014, -30.1604) -> (76.8126, -29.609)
  arc A47 (76.3649, -28.5856) -> (76.8126, -29.609) centre (77.1055, -28.8713) ccw
  arc A48 (76.3649, -28.5856) -> (78.0563, -23.7518) centre (0.5538, 0.6546) ccw
  arc A49 (79.0444, -23.2308) -> (78.0563, -23.7518) centre (78.8134, -23.9902) ccw
  line L22 (79.0444, -23.2308) -> (80.474, -23.6657)
  spline S22 degree 5 poles (80.474, -23.6657) (80.5071, -23.6757) (80.5736, -23.6951) (80.6739, -23.7216) (80.8087, -23.7524) (80.9787, -23.7846) (81.1499, -23.8122) (81.3217, -23.8371) (81.4939, -23.8604) (81.6663, -23.8828) (81.839, -23.904) (82.0119, -23.9238) (82.1852, -23.9417) (82.359, -23.9575) (82.5332, -23.9709) (82.7078, -23.9824) (82.8828, -23.9921) (83.058, -24.0003) (83.2334, -24.0073) (83.409, -24.0131) (83.5848, -24.0177) (83.7608, -24.021) (83.937, -24.0229) (84.1134, -24.0235) (84.2901, -24.0227) (84.4669, -24.0206) (84.6439, -24.0173) (84.821, -24.0128) (84.9983, -24.0072) (85.1757, -24.0005) (85.3533, -23.9926) (85.531, -23.9837) (85.7088, -23.9737) (85.8867, -23.9626) (86.0647, -23.9504) (86.2429, -23.9371) (86.4212, -23.9228) (86.5995, -23.9074) (86.7779, -23.8911) (86.9565, -23.8738) (87.1351, -23.8554) (87.3138, -23.8361) (87.4925, -23.8159) (87.6714, -23.7947) (87.8503, -23.7725) (88.0292, -23.7494) (88.2082, -23.7253) (88.3873, -23.7003) (88.5664, -23.6745) (88.7456, -23.6477) (88.9248, -23.62) (89.104, -23.5914) (89.2833, -23.562) (89.4626, -23.5316) (89.642, -23.5004) (89.8213, -23.4684) (90.0007, -23.4355) (90.1801, -23.4017) (90.3596, -23.3671) (90.539, -23.3316) (90.7185, -23.2953) (90.8979, -23.2582) (91.0774, -23.2203) (91.2568, -23.1815) (91.4363, -23.142) (91.6158, -23.1016) (91.7952, -23.0605) (91.9747, -23.0185) (92.1541, -22.9758) (92.3336, -22.9322) (92.513, -22.8879) (92.6565, -22.8519) (92.7641, -22.8245) (92.8359, -22.806) (92.8717, -22.7968) knots 0 0 0 0 0 0 0.01428571 0.02857143 0.04285714 0.05714286 0.07142857 0.08571429 0.1 0.11428571 0.12857143 0.14285714 0.15714286 0.17142857 0.18571429 0.2 0.21428571 0.22857143 0.24285714 0.25714286 0.27142857 0.28571429 0.3 0.31428571 0.32857143 0.34285714 0.35714286 0.37142857 0.38571429 0.4 0.41428571 0.42857143 0.44285714 0.45714286 0.47142857 0.48571429 0.5 0.51428571 0.52857143 0.54285714 0.55714286 0.57142857 0.58571429 0.6 0.61428571 0.62857143 0.64285714 0.65714286 0.67142857 0.68571429 0.7 0.71428571 0.72857143 0.74285714 0.75714286 0.77142857 0.78571429 0.8 0.81428571 0.82857143 0.84285714 0.85714286 0.87142857 0.88571429 0.9 0.91428571 0.92857143 0.94285714 0.95714286 0.97142857 0.98571429 1 1 1 1 1 1
  arc A50 (92.8717, -22.7968) -> (93.9046, -18.2716) centre (0.5538, 0.6546) ccw
  spline S23 degree 5 poles (83.1116, -12.1096) (83.1458, -12.1149) (83.2141, -12.1263) (83.316, -12.1459) (83.4508, -12.1766) (83.618, -12.2214) (83.7842, -12.2708) (83.9497, -12.3229) (84.115, -12.3766) (84.28, -12.4313) (84.4448, -12.4871) (84.6092, -12.5442) (84.7731, -12.6033) (84.9365, -12.6646) (85.0993, -12.728) (85.2616, -12.7934) (85.4235, -12.8606) (85.5849, -12.9292) (85.746, -12.999) (85.9067, -13.07) (86.0671, -13.1422) (86.2271, -13.2156) (86.3867, -13.2903) (86.5459, -13.3663) (86.7047, -13.4436) (86.8631, -13.5222) (87.0211, -13.602) (87.1788, -13.6829) (87.336, -13.7649) (87.493, -13.8479) (87.6495, -13.932) (87.8058, -14.0172) (87.9616, -14.1033) (88.1171, -14.1906) (88.2722, -14.2788) (88.427, -14.3681) (88.5814, -14.4583) (88.7354, -14.5495) (88.8891, -14.6417) (89.0424, -14.7347) (89.1954, -14.8287) (89.348, -14.9236) (89.5003, -15.0195) (89.6522, -15.1162) (89.8037, -15.2138) (89.9549, -15.3123) (90.1058, -15.4116) (90.2563, -15.5118) (90.4064, -15.6128) (90.5562, -15.7147) (90.7057, -15.8174) (90.8548, -15.9209) (91.0035, -16.0252) (91.1519, -16.1304) (91.3, -16.2363) (91.4477, -16.343) (91.595, -16.4505) (91.742, -16.5588) (91.8886, -16.6678) (92.0349, -16.7776) (92.1809, -16.8881) (92.3264, -16.9994) (92.4717, -17.1115) (92.6166, -17.2243) (92.7611, -17.3378) (92.9053, -17.452) (93.0491, -17.5669) (93.1926, -17.6826) (93.3357, -17.799) (93.4785, -17.916) (93.6209, -18.0338) (93.7345, -18.1286) (93.8196, -18.2) (93.8763, -18.2477) (93.9046, -18.2716) knots 0 0 0 0 0 0 0.01428571 0.02857143 0.04285714 0.05714286 0.07142857 0.08571429 0.1 0.11428571 0.12857143 0.14285714 0.15714286 0.17142857 0.18571429 0.2 0.21428571 0.22857143 0.24285714 0.25714286 0.27142857 0.28571429 0.3 0.31428571 0.32857143 0.34285714 0.35714286 0.37142857 0.38571429 0.4 0.41428571 0.42857143 0.44285714 0.45714286 0.47142857 0.48571429 0.5 0.51428571 0.52857143 0.54285714 0.55714286 0.57142857 0.58571429 0.6 0.61428571 0.62857143 0.64285714 0.65714286 0.67142857 0.68571429 0.7 0.71428571 0.72857143 0.74285714 0.75714286 0.77142857 0.78571429 0.8 0.81428571 0.82857143 0.84285714 0.85714286 0.87142857 0.88571429 0.9 0.91428571 0.92857143 0.94285714 0.95714286 0.97142857 0.98571429 1 1 1 1 1 1
  line L23 (83.1116, -12.1096) -> (81.6349, -11.8811)
  arc A51 (80.9707, -10.983) -> (81.6349, -11.8811) centre (81.7563, -11.0966) ccw
  arc A52 (80.9707, -10.983) -> (81.5441, -5.894) centre (0.5538, 0.6546) ccw
  arc A53 (82.3915, -5.1662) -> (81.5441, -5.894) centre (82.3353, -5.958) ccw
  line L24 (82.3915, -5.1662) -> (83.882, -5.272)
  spline S24 degree 5 poles (83.882, -5.272) (83.9166, -5.2744) (83.9856, -5.2785) (84.0893, -5.2821) (84.2276, -5.2821) (84.4006, -5.2756) (84.5736, -5.2645) (84.7466, -5.2505) (84.9197, -5.2349) (85.0927, -5.2183) (85.2658, -5.2006) (85.4388, -5.1815) (85.6118, -5.1604) (85.7847, -5.137) (85.9575, -5.1114) (86.1303, -5.0837) (86.303, -5.0542) (86.4757, -5.0233) (86.6483, -4.991) (86.8208, -4.9576) (86.9932, -4.9229) (87.1655, -4.887) (87.3377, -4.8497) (87.5098, -4.811) (87.6819, -4.7709) (87.8538, -4.7296) (88.0256, -4.6869) (88.1973, -4.6431) (88.3689, -4.5982) (88.5404, -4.5522) (88.7117, -4.505) (88.883, -4.4568) (89.0541, -4.4075) (89.2251, -4.357) (89.3959, -4.3055) (89.5667, -4.2529) (89.7373, -4.1993) (89.9077, -4.1446) (90.0781, -4.089) (90.2483, -4.0324) (90.4183, -3.9748) (90.5882, -3.9162) (90.758, -3.8567) (90.9276, -3.7962) (91.0971, -3.7348) (91.2664, -3.6724) (91.4356, -3.6091) (91.6046, -3.5449) (91.7735, -3.4798) (91.9422, -3.4139) (92.1108, -3.347) (92.2792, -3.2793) (92.4474, -3.2106) (92.6155, -3.1412) (92.7834, -3.0708) (92.9511, -2.9997) (93.1187, -2.9277) (93.2861, -2.8548) (93.4533, -2.7811) (93.6203, -2.7067) (93.7872, -2.6313) (93.9539, -2.5552) (94.1204, -2.4783) (94.2868, -2.4006) (94.453, -2.3221) (94.6189, -2.2428) (94.7847, -2.1628) (94.9504, -2.0819) (95.1158, -2.0003) (95.281, -1.918) (95.4461, -1.8348) (95.578, -1.7677) (95.6768, -1.7171) (95.7426, -1.6831) (95.7756, -1.6661) knots 0 0 0 0 0 0 0.01428571 0.02857143 0.04285714 0.05714286 0.07142857 0.08571429 0.1 0.11428571 0.12857143 0.14285714 0.15714286 0.17142857 0.18571429 0.2 0.21428571 0.22857143 0.24285714 0.25714286 0.27142857 0.28571429 0.3 0.31428571 0.32857143 0.34285714 0.35714286 0.37142857 0.38571429 0.4 0.41428571 0.42857143 0.44285714 0.45714286 0.47142857 0.48571429 0.5 0.51428571 0.52857143 0.54285714 0.55714286 0.57142857 0.58571429 0.6 0.61428571 0.62857143 0.64285714 0.65714286 0.67142857 0.68571429 0.7 0.71428571 0.72857143 0.74285714 0.75714286 0.77142857 0.78571429 0.8 0.81428571 0.82857143 0.84285714 0.85714286 0.87142857 0.88571429 0.9 0.91428571 0.92857143 0.94285714 0.95714286 0.97142857 0.98571429 1 1 1 1 1 1
  arc A54 (95.7756, -1.6661) -> (95.7756, 2.9754) centre (0.5538, 0.6546) ccw
  spline S25 degree 5 poles (83.882, 6.5813) (83.9166, 6.5837) (83.9856, 6.5878) (84.0893, 6.5914) (84.2276, 6.5914) (84.4006, 6.5849) (84.5736, 6.5738) (84.7466, 6.5598) (84.9197, 6.5442) (85.0927, 6.5276) (85.2658, 6.5099) (85.4388, 6.4908) (85.6118, 6.4697) (85.7847, 6.4463) (85.9575, 6.4207) (86.1303, 6.393) (86.303, 6.3635) (86.4757, 6.3326) (86.6483, 6.3003) (86.8208, 6.2669) (86.9932, 6.2322) (87.1655, 6.1963) (87.3377, 6.159) (87.5098, 6.1203) (87.6819, 6.0802) (87.8538, 6.0388) (88.0256, 5.9962) (88.1973, 5.9524) (88.3689, 5.9075) (88.5404, 5.8615) (88.7117, 5.8143) (88.883, 5.7661) (89.0541, 5.7167) (89.2251, 5.6663) (89.3959, 5.6148) (89.5667, 5.5622) (89.7373, 5.5086) (89.9077, 5.4539) (90.0781, 5.3983) (90.2483, 5.3417) (90.4183, 5.2841) (90.5882, 5.2255) (90.758, 5.166) (90.9276, 5.1055) (91.0971, 5.044) (91.2664, 4.9817) (91.4356, 4.9184) (91.6046, 4.8542) (91.7735, 4.7891) (91.9422, 4.7231) (92.1108, 4.6563) (92.2792, 4.5885) (92.4474, 4.5199) (92.6155, 4.4504) (92.7834, 4.3801) (92.9511, 4.3089) (93.1187, 4.2369) (93.2861, 4.1641) (93.4533, 4.0904) (93.6203, 4.0159) (93.7872, 3.9406) (93.9539, 3.8645) (94.1204, 3.7876) (94.2868, 3.7099) (94.453, 3.6314) (94.6189, 3.5521) (94.7847, 3.472) (94.9504, 3.3912) (95.1158, 3.3096) (95.281, 3.2272) (95.4461, 3.1441) (95.578, 3.077) (95.6768, 3.0263) (95.7426, 2.9924) (95.7756, 2.9754) knots 0 0 0 0 0 0 0.01428571 0.02857143 0.04285714 0.05714286 0.07142857 0.08571429 0.1 0.11428571 0.12857143 0.14285714 0.15714286 0.17142857 0.18571429 0.2 0.21428571 0.22857143 0.24285714 0.25714286 0.27142857 0.28571429 0.3 0.31428571 0.32857143 0.34285714 0.35714286 0.37142857 0.38571429 0.4 0.41428571 0.42857143 0.44285714 0.45714286 0.47142857 0.48571429 0.5 0.51428571 0.52857143 0.54285714 0.55714286 0.57142857 0.58571429 0.6 0.61428571 0.62857143 0.64285714 0.65714286 0.67142857 0.68571429 0.7 0.71428571 0.72857143 0.74285714 0.75714286 0.77142857 0.78571429 0.8 0.81428571 0.82857143 0.84285714 0.85714286 0.87142857 0.88571429 0.9 0.91428571 0.92857143 0.94285714 0.95714286 0.97142857 0.98571429 1 1 1 1 1 1
  line L25 (83.882, 6.5813) -> (82.3915, 6.4755)
  arc A55 (81.5441, 7.2033) -> (82.3915, 6.4755) centre (82.3353, 7.2672) ccw
  arc A56 (81.5441, 7.2033) -> (80.9707, 12.2922) centre (0.5538, 0.6546) ccw
  arc A57 (81.6349, 13.1903) -> (80.9707, 12.2922) centre (81.7563, 12.4059) ccw
  line L26 (81.6349, 13.1903) -> (83.1116, 13.4189)
  spline S26 degree 5 poles (83.1116, 13.4189) (83.1458, 13.4242) (83.2141, 13.4356) (83.316, 13.4551) (83.4508, 13.4859) (83.618, 13.5307) (83.7842, 13.5801) (83.9497, 13.6322) (84.115, 13.6859) (84.28, 13.7406) (84.4448, 13.7963) (84.6092, 13.8535) (84.7731, 13.9126) (84.9365, 13.9738) (85.0993, 14.0373) (85.2616, 14.1027) (85.4235, 14.1699) (85.5849, 14.2385) (85.746, 14.3083) (85.9067, 14.3793) (86.0671, 14.4515) (86.2271, 14.5248) (86.3867, 14.5995) (86.5459, 14.6756) (86.7047, 14.7529) (86.8631, 14.8315) (87.0211, 14.9113) (87.1788, 14.9922) (87.336, 15.0742) (87.493, 15.1572) (87.6495, 15.2413) (87.8058, 15.3264) (87.9616, 15.4126) (88.1171, 15.4998) (88.2722, 15.5881) (88.427, 15.6774) (88.5814, 15.7676) (88.7354, 15.8588) (88.8891, 15.9509) (89.0424, 16.044) (89.1954, 16.138) (89.348, 16.2329) (89.5003, 16.3287) (89.6522, 16.4255) (89.8037, 16.5231) (89.9549, 16.6215) (90.1058, 16.7209) (90.2563, 16.8211) (90.4064, 16.9221) (90.5562, 17.024) (90.7057, 17.1267) (90.8548, 17.2302) (91.0035, 17.3345) (91.1519, 17.4396) (91.3, 17.5456) (91.4477, 17.6523) (91.595, 17.7598) (91.742, 17.868) (91.8886, 17.9771) (92.0349, 18.0869) (92.1809, 18.1974) (92.3264, 18.3087) (92.4717, 18.4208) (92.6166, 18.5335) (92.7611, 18.647) (92.9053, 18.7613) (93.0491, 18.8762) (93.1926, 18.9919) (93.3357, 19.1082) (93.4785, 19.2253) (93.6209, 19.3431) (93.7345, 19.4379) (93.8196, 19.5092) (93.8763, 19.557) (93.9046, 19.5809) knots 0 0 0 0 0 0 0.01428571 0.02857143 0.04285714 0.05714286 0.07142857 0.08571429 0.1 0.11428571 0.12857143 0.14285714 0.15714286 0.17142857 0.18571429 0.2 0.21428571 0.22857143 0.24285714 0.25714286 0.27142857 0.28571429 0.3 0.31428571 0.32857143 0.34285714 0.35714286 0.37142857 0.38571429 0.4 0.41428571 0.42857143 0.44285714 0.45714286 0.47142857 0.48571429 0.5 0.51428571 0.52857143 0.54285714 0.55714286 0.57142857 0.58571429 0.6 0.61428571 0.62857143 0.64285714 0.65714286 0.67142857 0.68571429 0.7 0.71428571 0.72857143 0.74285714 0.75714286 0.77142857 0.78571429 0.8 0.81428571 0.82857143 0.84285714 0.85714286 0.87142857 0.88571429 0.9 0.91428571 0.92857143 0.94285714 0.95714286 0.97142857 0.98571429 1 1 1 1 1 1
  arc A58 (93.9046, 19.5809) -> (92.8717, 24.1061) centre (0.5538, 0.6546) ccw
  spline S27 degree 5 poles (80.474, 24.9749) (80.5071, 24.985) (80.5736, 25.0043) (80.6739, 25.0309) (80.8087, 25.0617) (80.9787, 25.0939) (81.1499, 25.1215) (81.3217, 25.1464) (81.4939, 25.1697) (81.6663, 25.192) (81.839, 25.2133) (82.0119, 25.2331) (82.1852, 25.251) (82.359, 25.2667) (82.5332, 25.2802) (82.7078, 25.2917) (82.8828, 25.3014) (83.058, 25.3096) (83.2334, 25.3166) (83.409, 25.3224) (83.5848, 25.3269) (83.7608, 25.3302) (83.937, 25.3322) (84.1134, 25.3328) (84.2901, 25.332) (84.4669, 25.3299) (84.6439, 25.3266) (84.821, 25.3221) (84.9983, 25.3165) (85.1757, 25.3097) (85.3533, 25.3019) (85.531, 25.293) (85.7088, 25.283) (85.8867, 25.2718) (86.0647, 25.2596) (86.2429, 25.2464) (86.4212, 25.232) (86.5995, 25.2167) (86.7779, 25.2004) (86.9565, 25.183) (87.1351, 25.1647) (87.3138, 25.1454) (87.4925, 25.1252) (87.6714, 25.1039) (87.8503, 25.0818) (88.0292, 25.0586) (88.2082, 25.0346) (88.3873, 25.0096) (88.5664, 24.9837) (88.7456, 24.957) (88.9248, 24.9293) (89.104, 24.9007) (89.2833, 24.8712) (89.4626, 24.8409) (89.642, 24.8097) (89.8213, 24.7777) (90.0007, 24.7447) (90.1801, 24.711) (90.3596, 24.6763) (90.539, 24.6409) (90.7185, 24.6046) (90.8979, 24.5675) (91.0774, 24.5296) (91.2568, 24.4908) (91.4363, 24.4513) (91.6158, 24.4109) (91.7952, 24.3697) (91.9747, 24.3278) (92.1541, 24.2851) (92.3336, 24.2415) (92.513, 24.1972) (92.6565, 24.1611) (92.7641, 24.1337) (92.8359, 24.1153) (92.8717, 24.1061) knots 0 0 0 0 0 0 0.01428571 0.02857143 0.04285714 0.05714286 0.07142857 0.08571429 0.1 0.11428571 0.12857143 0.14285714 0.15714286 0.17142857 0.18571429 0.2 0.21428571 0.22857143 0.24285714 0.25714286 0.27142857 0.28571429 0.3 0.31428571 0.32857143 0.34285714 0.35714286 0.37142857 0.38571429 0.4 0.41428571 0.42857143 0.44285714 0.45714286 0.47142857 0.48571429 0.5 0.51428571 0.52857143 0.54285714 0.55714286 0.57142857 0.58571429 0.6 0.61428571 0.62857143 0.64285714 0.65714286 0.67142857 0.68571429 0.7 0.71428571 0.72857143 0.74285714 0.75714286 0.77142857 0.78571429 0.8 0.81428571 0.82857143 0.84285714 0.85714286 0.87142857 0.88571429 0.9 0.91428571 0.92857143 0.94285714 0.95714286 0.97142857 0.98571429 1 1 1 1 1 1
  line L27 (80.474, 24.9749) -> (79.0444, 24.5401)
  arc A59 (78.0563, 25.0611) -> (79.0444, 24.5401) centre (78.8134, 25.2995) ccw
  arc A60 (78.0563, 25.0611) -> (76.3649, 29.8949) centre (0.5538, 0.6546) ccw
  arc A61 (76.8126, 30.9183) -> (76.3649, 29.8949) centre (77.1055, 30.1805) ccw
  line L28 (76.8126, 30.9183) -> (78.2014, 31.4697)